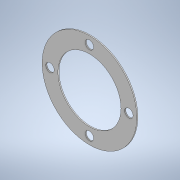
# Autodesk Inventor part: Part8
Saved by Autodesk Inventor 2021 (Build 250183000, 183)
## iProperties
Created: 2022-06-05
Part Number: Part8
Material: Generic
Document SubType Name: Modeling
Designer: Bhargav Malasani
Density: 1 g/cm^3
Appearance: Default
Author: Bhargav Malasani
Autodesk Inventor part; units mm, degrees
ref_plane "YZ Plane" through (0, 0, 0) normal (1, 0, 0) x (0, 1, 0)
ref_plane "XZ Plane" through (0, 0, 0) normal (0, 1, 0) x (-1, 0, 0)
ref_plane "XY Plane" through (0, 0, 0) normal (0, 0, 1) x (1, 0, 0)
sketch "Sketch1" plane through (0, 0, 0) normal (0, 0, 1) x (1, 0, 0)
  circle A0 centre (0, 0) radius 45
  circle A1 centre (0, 0) radius 30
  circle A2 centre (0, 37.5) radius 4
  circle A3 centre (-37.5, 0) radius 4
  circle A4 centre (0, -37.5) radius 4
  circle A5 centre (37.5, 0) radius 4
  dimension "d0" = 90
  dimension "d1" = 60
  dimension "d2" = 8
  dimension "d3" = 37.5
  dimension "d6" = 360
  dimension "d8" = 75
  dimension "d9" = 37.5
  dimension "d10" = 37.5
  dimension "d11" = 75
  constraints: 6 centre point, 2 coincident, 9 other
  measures "d0" diameter of A0
  measures "d1" diameter of A1
  measures "d2" diameter of A2
  measures "d3" distance of A2.centre point (0, 0)
  measures "d8" distance between centres of A4 A2
  measures "d9" distance of point (0, 0) A4.centre
  measures "d10" distance of point (0, 0) A3.centre
  measures "d11" distance of A5.centre A3.centre
extrude "Extrusion1" add sketch "Sketch1" along normal mid plane 1
body "Solid1"
